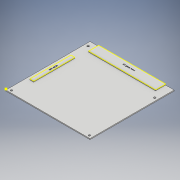
# Autodesk Inventor part: mini itx motherboard
Saved by Autodesk Inventor 2018 (Build 220112000, 112)
## iProperties
Created: 2018-06-06
Part Number: mini itx motherboard
Material: Generic
Document SubType Name: Modeling
Designer: John Viljoen
Density: 1 g/cm^3
Appearance: Default
Author: John Viljoen
Autodesk Inventor part; units mm, degrees
ref_plane "YZ Plane" through (0, 0, 0) normal (1, 0, 0) x (0, 1, 0)
ref_plane "XZ Plane" through (0, 0, 0) normal (0, 1, 0) x (-1, 0, 0)
ref_plane "XY Plane" through (0, 0, 0) normal (0, 0, 1) x (1, 0, 0)
sketch "Sketch1" plane through (0, 0, 0) normal (0, 0, 1) x (1, 0, 0)
  line L0 (0, 0) -> (170, 0)
  line L1 (170, 0) -> (170, 170)
  line L2 (170, 170) -> (0, 170)
  line L3 (0, 170) -> (0, 0)
  dimension "d0" = 170
  dimension "d1" = 170
  constraints: 8 end point, 2 parallel, 1 horizontal, 1 perpendicular
  measures "d0" distance of L2.end L1.end
  measures "d1" distance of L1.end L0.end
extrude "Extrusion1" add sketch "Sketch1" along normal blind 2
sketch "Sketch2" plane through (0, 0, 2) normal (0, 0, 1) x (1, 0, 0)
  line L0 (170, 170) -> (0, 170) projected
  line L1 (0, 170) -> (0, 0) projected
  line L2 (0, 170) -> (0, 159.84) construction
  line L3 (0, 159.84) -> (6.35, 159.84) construction
  line L4 (6.35, 170) -> (163.83, 170) construction
  line L5 (163.83, 170) -> (163.83, 136.98) construction
  line L6 (6.35, 159.84) -> (6.35, 4.9) construction
  line L7 (6.35, 4.9) -> (163.83, 4.9) construction
  circle A0 centre (6.35, 159.84) radius 1.98
  circle A1 centre (163.83, 136.98) radius 1.98
  circle A2 centre (6.35, 4.9) radius 1.98
  circle A3 centre (163.83, 4.9) radius 1.98
  dimension "d4" = 10.16
  dimension "d5" = 6.35
  dimension "d6" = 157.48
  dimension "d7" = 33.02
  dimension "d8" = 154.94
  dimension "d9" = 3.96
  dimension "d10" = 3.96
  dimension "d11" = 3.96
  dimension "d12" = 3.96
  constraints: 12 end point, 4 centre point, 4 coincident, 3 perpendicular, 3 point on line, 1 vertical
  measures "d4" distance of L0.end L2.end
  measures "d5" distance of L2.end L3.end
  measures "d6" distance of L4.start L4.end
  measures "d7" distance of L4.end L5.end
  measures "d8" distance of L3.end L6.end
  measures "d9" diameter of A0
  measures "d10" diameter of A1
  measures "d11" diameter of A2
  measures "d12" diameter of A3
extrude "Extrusion2" cut sketch "Sketch2" against normal blind 2
sketch "Sketch3" plane through (0, 0, 2) normal (0, 0, 1) x (1, 0, 0)
  line L0 (14.2327, 124.8626) -> (6.35, 124.8626)
  line L1 (6.35, 124.8626) -> (6.35, 41.7782)
  line L2 (6.35, 41.7782) -> (14.2327, 41.7782)
  line L3 (14.2327, 41.7782) -> (14.2327, 124.8626)
  constraints: 8 end point, 2 parallel, 1 horizontal, 1 perpendicular
extrude "Extrusion3" add sketch "Sketch3" along normal blind 2
sketch "Sketch4" plane through (0, 0, 4) normal (0, 0, 1) x (1, 0, 0)
  line L0 (14.2327, 124.8626) -> (6.35, 124.8626) projected
  line L1 (6.35, 124.8626) -> (6.35, 41.7782) projected
  line L2 (6.35, 41.7782) -> (14.2327, 41.7782) projected
  line L3 (14.2327, 41.7782) -> (14.2327, 124.8626) projected
  line L4 (12.3491, 93.2345) -> (12.3491, 74.2867) construction
  line L5 (12.3491, 74.2867) -> (8.2093, 74.2867) construction
  line L6 (8.2093, 74.2867) -> (8.2093, 93.2345) construction
  line L7 (8.2093, 93.2345) -> (12.3491, 93.2345) construction
  point P0 (0, 0)
  constraints: 2 other
sketch "Sketch5" plane through (0, 0, 2) normal (0, 0, 1) x (1, 0, 0)
  line L0 (170, 170) -> (0, 170) projected
  line L1 (17.1297, 170) -> (152.7432, 170)
  line L2 (152.7432, 170) -> (152.7432, 149.8199)
  line L3 (152.7432, 149.8199) -> (17.1297, 149.8199)
  line L4 (17.1297, 149.8199) -> (17.1297, 170)
  constraints: 8 end point, 2 parallel, 1 horizontal, 1 perpendicular, 1 point on line
extrude "Extrusion4" add sketch "Sketch5" along normal blind 2
sketch "Sketch6" plane through (0, 0, 4) normal (0, 0, 1) x (1, 0, 0)
  line L0 (17.1297, 170) -> (17.1297, 149.8199) projected
  line L1 (17.1297, 149.8199) -> (152.7432, 149.8199) projected
  line L2 (152.7432, 149.8199) -> (152.7432, 170) projected
  line L3 (152.7432, 170) -> (17.1297, 170) projected
  line L4 (74.7193, 163.8007) -> (99.6305, 163.8007) construction
  line L5 (99.6305, 163.8007) -> (99.6305, 158.8439) construction
  line L6 (99.6305, 158.8439) -> (74.7193, 158.8439) construction
  line L7 (74.7193, 158.8439) -> (74.7193, 163.8007) construction
  point P0 (0, 0)
  constraints: 2 other
body "Solid1"
